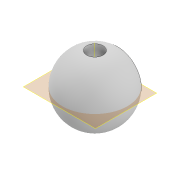
# Autodesk Inventor part: HeadP
Saved by Autodesk Inventor 2021 (Build 250183000, 183)
## iProperties
Created: 2020-12-19
Part Number: HeadP
Material: 一般
Document SubType Name: Modeling
Designer: Tazaki
Density: 0.563797 g/cm^3
Appearance: 既定
Mass: 2000 g
Surface Area: 1492.59 cm^2
Volume: 3547.38 cm^3
Author: Tazaki
Autodesk Inventor part; units mm, degrees
ref_plane "YZ Plane" through (0, 0, 0) normal (1, 0, 0) x (0, 1, 0)
ref_plane "XY Plane" through (0, 0, 0) normal (0, 0, 1) x (1, 0, 0)
sketch "スケッチ1" plane through (0, 0, 0) normal (0, 0, 1) x (1, 0, 0)
  arc A0 (0, 100) -> (0, -100) centre (0, 0) ccw
  line L0 (0, 100) -> (0, -100)
  dimension "d0" = 200
  constraints: 2 end point, 2 point on circle, 1 centre point, 1 coincident, 1 vertical
  measures "d0" diameter of A0
revolve "回転1" add sketch "スケッチ1" angle 360 about axis through (0, 100, 0) along (0, -1, 0)
sketch "スケッチ2" plane through (0, 0, 0) normal (0, 1, 0) x (-1, 0, 0)
  line L0 (140.6562, -148.6683) -> (-138.1636, -148.6683)
  line L1 (-138.1636, -148.6683) -> (-138.1636, -69.972)
  line L2 (-138.1636, -69.972) -> (140.6562, -69.972)
  line L3 (140.6562, -69.972) -> (140.6562, -148.6683)
  point P0 (0, 0)
  constraints: 8 end point, 2 parallel, 1 horizontal, 1 perpendicular
extrude "押し出し1" cut sketch "スケッチ2" along normal mid plane 200
sketch "スケッチ3" plane through (0, 0, 0) normal (0, 1, 0) x (-1, 0, 0)
  circle A0 centre (0, 0) radius 25
  dimension "d4" = 50
  constraints: 1 centre point, 1 coincident
  measures "d4" diameter of A0
extrude "押し出し2" cut sketch "スケッチ3" along normal mid plane 200
